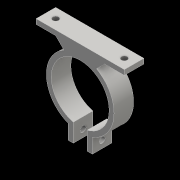
# Autodesk Inventor part: pumpholder
Saved by Autodesk Inventor 2016 (Build 200138000, 138)
## iProperties
Created: 2019-01-16
Part Number: pumpholder
Material: Generic
Document SubType Name: Modeling
Designer: Calb3
Density: 1 g/cm^3
Appearance: Default
Author: Calb3
Autodesk Inventor part; units mm, degrees
ref_plane "YZ Plane" through (0, 0, 0) normal (1, 0, 0) x (0, 1, 0)
ref_plane "XZ Plane" through (0, 0, 0) normal (0, 1, 0) x (-1, 0, 0)
ref_plane "XY Plane" through (0, 0, 0) normal (0, 0, 1) x (1, 0, 0)
sketch "Sketch1" plane through (0, 0, 0) normal (0, 1, 0) x (-1, 0, 0)
  arc A0 (7, -28.6575) -> (-7, -28.6575) centre (0, 0) ccw
  arc A1 (12.4228, -32.1858) -> (-12.4228, -32.1858) centre (0, 0) ccw
  line L0 (16.5147, 30.2905) -> (25, 38.7758)
  line L1 (16.5147, 30.2905) -> (28.5147, 30.2905) construction
  line L2 (25, 38.7758) -> (-25, 38.7758)
  line L3 (-25, 38.7758) -> (-16.5147, 30.2905)
  line L4 (12.4228, -32.1858) -> (12.4228, -47.1858)
  line L5 (12.4228, -47.1858) -> (7, -47.1858)
  line L6 (7, -47.1858) -> (7, -28.6575)
  line L7 (0, 0) -> (0, -37.5587) construction
  line L8 (-12.4228, -32.1858) -> (-12.4228, -47.1858)
  line L9 (-12.4228, -47.1858) -> (-7, -47.1858)
  line L10 (-7, -47.1858) -> (-7, -28.6575)
  dimension "d0" = 59
  dimension "d5" = 12
  dimension "d6" = 45
  dimension "d7" = 5
  dimension "d15" = 15
  dimension "d46" = 50
  dimension "d47" = 45
  dimension "d48" = 5.4228
  dimension "d49" = 14
  dimension "d50" = 12
  constraints: 22 end point, 6 point on circle, 3 horizontal, 3 vertical, 2 centre point, 2 symmetric about line, 1 coincident, 1 equal length, 1 perpendicular
  measures "d0" diameter of A0
  measures "d5" distance of L0.start L0.end
  measures "d6" angle of L1 L0
  measures "d7" radial gap between concentric circles of A1 A0
  measures "d15" distance of L4.start L4.end
  measures "d46" distance of L0.end L2.end
  measures "d47" angle of L2 L3
  measures "d48" distance between parallel lines of L4 L6
  measures "d49" distance between parallel lines of L10 L6
  measures "d50" distance of L2.end L3.end
extrude "Extrusion3" add sketch "Sketch1" along normal blind 20
sketch "Sketch3" plane through (-25, 0, 38.7758) normal (0, 0, 1) x (1, 0, 0)
  line L0 (0, 0) -> (50, 0) projected
  line L1 (0, 20) -> (50, 20) projected
  line L2 (-20, 0) -> (70, 0)
  line L3 (70, 0) -> (70, 20)
  line L4 (70, 20) -> (-20, 20)
  line L5 (-20, 20) -> (-20, 0)
  point P0 (25, 0)
  point P1 (25, 20)
  dimension "d18" = 90
  dimension "d19" = 20
  constraints: 8 end point, 2 midpoint, 2 parallel, 1 horizontal, 1 perpendicular
  measures "d18" distance of L2.start L2.end
  measures "d19" distance of L4.end L2.start
extrude "Extrusion4" add sketch "Sketch3" along normal blind 5
hole "Hole3" at (-12.4228, 10, -39.6858) direction (1, 0, 0) diameter 6 end through all
hole "Hole4" at (-35, 10, 38.7758) direction (0, 0, 1) diameter 6 end through all
hole "Hole5" at (35, 10, 38.7758) direction (0, 0, 1) diameter 6 end through all
body "Solid3"
